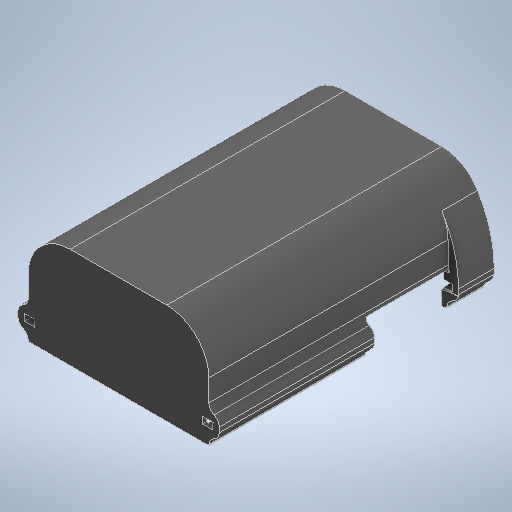
# Autodesk Inventor part: back_battery_case
Saved by Autodesk Inventor 2026.1 (Build 301233020, 233B)
## iProperties
Created: 2026-02-05
Part Number: back_battery_case
Material: 一般
Document SubType Name: Modeling
Designer: hibik
Density: 1 g/cm^3
Appearance: 既定
Author: hibik
Autodesk Inventor part; units mm, degrees
ref_plane "YZ Plane" through (0, 0, 0) normal (1, 0, 0) x (0, 1, 0)
ref_plane "XZ Plane" through (0, 0, 0) normal (0, 1, 0) x (-1, 0, 0)
ref_plane "XY Plane" through (0, 0, 0) normal (0, 0, 1) x (1, 0, 0)
sketch "スケッチ1" plane through (0, 0, 0) normal (0, 0, 1) x (1, 0, 0)
  line L0 (-20.5, 0) -> (20.5, 0)
  line L1 (20.5, 0) -> (20.5, 23)
  line L2 (20.5, 23) -> (-20.5, 23)
  line L3 (-20.5, 23) -> (-20.5, 0)
  point P0 (0, 0)
  point P1 (0, 0)
  dimension "d0" = 41
  dimension "d1" = 23
  constraints: 8 end point, 2 parallel, 1 coincident, 1 horizontal, 1 midpoint, 1 perpendicular
  measures "d0" distance of L2.end L1.end
  measures "d1" distance of L1.end L0.end
extrude "押し出し1" add sketch "スケッチ1" along normal blind 64.5
shell "シェル1" thickness 1 outward yes removed faces 2 at (-6.8333, 15.3333, 0) at (-6.8333, 0, 21.5)
fillet "フィレット1" radius 10 4 edges at (-21.5, 24, 32.75) (-20.5, 23, 32.25) (20.5, 23, 32.25) (21.5, 24, 32.75)
sketch "スケッチ2" plane through (0, 0, 65.5) normal (0, 0, 1) x (1, 0, 0)
  line L0 (-18, -4) -> (-18, 0) projected
  line L1 (-18, 0) -> (18, 0) projected
  line L2 (18, 0) -> (18, -4) projected
  line L3 (20, -4) -> (18, -4) projected
  line L4 (20, 4) -> (20, -4) projected
  line L5 (22, 4) -> (20, 4) projected
  line L6 (22, 5) -> (22, 4) projected
  line L7 (20, 5) -> (22, 5) projected
  line L8 (20, 8) -> (20, 5) projected
  line L9 (-20, 8) -> (20, 8) projected
  line L10 (-20, 5) -> (-20, 8) projected
  line L11 (-22, 5) -> (-20, 5) projected
  line L12 (-22, 4) -> (-22, 5) projected
  line L13 (-20, 4) -> (-22, 4) projected
  line L14 (-20, -4) -> (-20, 4) projected
  line L15 (-18, -4) -> (-20, -4) projected
  line L16 (-22.5, 5.3) -> (-20, 5.3)
  line L17 (-20, 5.3) -> (-20, 3.7)
  line L18 (-20, 3.7) -> (-22.5, 3.7)
  line L19 (-22.5, 3.7) -> (-22.5, 5.3)
  line L20 (22.5, 5.3) -> (20, 5.3)
  line L21 (20, 5.3) -> (20, 3.7)
  line L22 (20, 3.7) -> (22.5, 3.7)
  line L23 (22.5, 3.7) -> (22.5, 5.3)
  point P0 (0, 0)
  point P1 (-22.5, 4.5)
  point P2 (-22, 4.5)
  point P3 (22, 4.5)
  point P4 (22.5, 4.5)
  dimension "d6" = 0.3
  dimension "d7" = 0.5
  constraints: 16 end point, 4 midpoint, 4 parallel, 4 point on line, 2 horizontal, 2 horizontal alignment, 2 perpendicular, 1 collinear
  measures "d6" distance between parallel lines of L16 L11
  measures "d7" distance between parallel lines of L19 L12
extrude "押し出し2" cut sketch "スケッチ2" against normal up to surface (65.5 mm away) contours L18 L19 L16 L10 L11 L12 L13 L14 | L13 L12 L11 L17 | L4 L5 L6 L7 L8 L20 L23 L22 | L21 L7 L6 L5
sketch "スケッチ3" plane through (0, 0, 65.5) normal (0, 0, 1) x (1, 0, 0)
  line L0 (20.5, 5.3) -> (20, 5.3) projected
  line L1 (20, 5.3) -> (22.5, 5.3)
  line L2 (22.5, 5.3) -> (22.5, 3.7)
  line L3 (22.5, 3.7) -> (20, 3.7)
  line L4 (20, 3.7) -> (20, 5.3)
  line L5 (21.5, 6.8) -> (24, 6.8)
  line L6 (24, 6.8) -> (24, 2.2)
  line L7 (24, 2.2) -> (21.5, 2.2)
  line L8 (21.5, 2.2) -> (21.5, 6.8)
  line L9 (22, 5) -> (22, 4) projected
  line L10 (21.5, 5.3) -> (21.5, 14) projected
  point P0 (0, 0)
  point P1 (22.5, 4.5)
  point P2 (24, 4.5)
  point P3 (21.5, 3.7)
  dimension "d10" = 0.5
  dimension "d11" = 1.5
  dimension "d12" = 1.5
  constraints: 16 end point, 4 parallel, 2 horizontal, 2 midpoint, 2 perpendicular, 1 horizontal alignment, 1 point on line
  measures "d10" distance between parallel lines of L9 L2
  measures "d11" distance between parallel lines of L6 L2
  measures "d12" distance between parallel lines of L5 L1
extrude "押し出し3" add sketch "スケッチ3" against normal up to surface (65.5 mm away) contours L8 L5 L6 L7 L3 L2 L1
mirror "ミラー1" about plane through (0, 0, 0) normal (1, 0, 0) of "押し出し3"
fillet "フィレット3" radius 2 8 edges at (-21.5, 6.8, 32.75) (-24, 6.8, 32.75) (-24, 2.2, 32.75) (-21.5, 2.2, 32.75) (24, 2.2, 32.75) (21.5, 2.2, 32.75) (24, 6.8, 32.75) (21.5, 6.8, 32.75)
sketch "スケッチ4" plane through (21.5, 14, 65.5) normal (1, 0, 0) x (0, 0, -1)
  line L0 (37.5, -10) -> (55.5, -10) projected
  line L1 (37.5, -7) -> (55.5, -7) projected
  line L2 (37.5, -7) -> (37.5, -10)
  line L3 (55.5, -10) -> (55.5, -7)
  line L4 (0, -10.3) -> (65.5, -10.3) projected
  line L5 (37, -6.5) -> (57, -6.5)
  line L6 (57, -6.5) -> (57, -10.5)
  line L7 (57, -10.5) -> (37, -10.5)
  line L8 (37, -10.5) -> (37, -6.5)
  point P0 (65.5, -14)
  point P1 (37.5, -8.5)
  point P2 (37, -8.5)
  dimension "d17" = 1.5
  dimension "d18" = 0.5
  dimension "d19" = 0.5
  constraints: 12 end point, 2 midpoint, 2 parallel, 2 perpendicular, 1 horizontal, 1 horizontal alignment, 1 vertical
  measures "d17" distance between parallel lines of L3 L6
  measures "d18" distance between parallel lines of L7 L0
  measures "d19" distance between parallel lines of L2 L8
extrude "押し出し4" cut sketch "スケッチ4" along normal through all both and the other way through all contours L2 L1 L3 L0 | L8 L5 L6 L4 | L4 L6 L7 L8
sketch "スケッチ5" plane through (-11.5, 24, 0) normal (0, 1, 0) x (1, 0, 0)
  line L0 (35.4579, -8.5) -> (35.4579, -28.5) projected
  arc A0 (35.4579, -8.5) -> (35.4579, -28.5) centre (35.4579, -18.5) ccw
  line L1 (-12.5, 0) -> (-12.5, -65.5) projected
  arc A1 (-12.5, -28.5) -> (-12.5, -8.5) centre (-12.5, -18.5) ccw
  line L2 (-11.25, -8.5) -> (-12.5, -8.5) projected
  point P0 (11.5, 0)
  dimension "d22" = 10
  constraints: 4 point on circle, 2 centre point, 2 point on line, 1 equal radius, 1 tangent
  measures "d22" radius of A0
sketch "スケッチ6" plane through (-21.5, 0, 65.5) normal (0, -1, 0) x (1, 0, 0)
  arc A0 (-2.5, -57) -> (-2.5, -37) centre (-2.5, -47) ccw projected
  line L0 (-2.5, -65.5) -> (-2.5, 0) projected
  arc A1 (45.4579, -37) -> (45.4579, -57) centre (45.4579, -47) ccw projected
  line L1 (45.4579, -57) -> (45.4579, -37) projected
  point P0 (21.5, -65.5)
extrude "押し出し5" cut sketch "スケッチ6" against normal blind 8
sketch "スケッチ7" plane through (0, 0, 0) normal (0, 0, -1) x (-1, 0, 0)
  arc A0 (-11.5, 24) -> (-21.5, 14) centre (-11.5, 14) ccw projected
  line L0 (-24, 5.0919) -> (-24, 3.9081) projected
  arc A1 (-20.0398, 19.2031) -> (-24, 5.0919) centre (3.1208, 5.0919) ccw
  line L1 (-24, 5.0919) -> (-24, 3.9081) projected
  arc A2 (24, 5.0919) -> (20.0398, 19.2031) centre (-3.1208, 5.0919) ccw
  arc A3 (21.5, 14) -> (11.5, 24) centre (11.5, 14) ccw projected
  line L2 (24, 5.0919) -> (24, 3.9081) projected
  line L3 (-21.5, 8.8) -> (-21.5, 14) projected
  arc A4 (-22.75, 6.946) -> (-21.5, 8.8) centre (-23.5, 8.8) ccw projected
  arc A5 (-22.75, 6.946) -> (-24, 5.0919) centre (-22, 5.0919) ccw projected
  line L4 (21.5, 14) -> (21.5, 8.8) projected
  arc A6 (21.5, 8.8) -> (22.75, 6.946) centre (23.5, 8.8) ccw projected
  arc A7 (24, 5.0919) -> (22.75, 6.946) centre (22, 5.0919) ccw projected
  point P0 (0, 0)
  constraints: 6 point on circle, 4 tangent, 2 centre point
extrude "押し出し6" add sketch "スケッチ7" against normal up to surface (8.5 mm away)
